Autodesk Fusion 360 part; units mm, degrees
(part 3 of 5)
extrude "Finger lift notch''''" cut sketch "草图17 (3)" along normal blind 4 bodies 10 in component "LS_RemovableGrate"
chamfer "R03 touch edge chamfer'''''''''" distance 0.4 angle 45 5 edges at (166.7, 184.65, 30) (110, 318.7, 30) (166.7, 279.35, 30) (110, 145.3, 30) (53.3, 232, 30) on bodies 10 in component "LS_RemovableGrate"
ref_plane "工作平面1" through (0, 0, 10) normal (0, 0, 1) x (1, 0, 0) in component "RS_Integrated"
sketch "草图1 (11)" plane through (0, 0, 10) normal (0, 0, 1) x (1, 0, 0) in component "RS_Integrated"
  line L0 (770, 142) -> (860, 142)
  line L1 (860, 142) -> (860, 322)
  line L2 (860, 322) -> (770, 322)
  line L3 (770, 322) -> (770, 142)
  dimension "d1020" = 770
  dimension "d1021" = 142
  dimension "d1022" = 90
  dimension "d1023" = 180
  constraint horizontal L0
  constraint vertical L1
  constraint horizontal L2
  constraint vertical L3
  measures "d1020" horizontal distance of origin L0.start
  measures "d1021" vertical distance of origin L0.start
  measures "d1022" horizontal distance of L0.start L0.end
  measures "d1023" vertical distance of L0.end L1.end
extrude "R04 pan blank'''''" add sketch "草图1 (11)" along normal blind 20 separate body makes body 11 in component "RS_Integrated"
fillet "Outside corner rounds'''''" radius 3 4 edges at (770, 322, 20) (860, 322, 20) (860, 142, 20) (770, 142, 20) on bodies 11 in component "RS_Integrated"
ref_plane "工作平面2" through (0, 145, 0) normal (0, 1, 0) x (0, 0, 1) in component "RS_Integrated"
sketch "草图2 (11)" plane through (0, 145, 0) normal (0, 1, 0) x (1, 0, 0) in component "RS_Integrated"
  line L0 (857, -22.1441) -> (770, -13)
  line L1 (770, -13) -> (770, -31)
  line L2 (770, -31) -> (857, -31)
  line L3 (857, -31) -> (857, -22.1441)
  dimension "d1030" = 857
  dimension "d1031" = 22.1441
  dimension "d1032" = 770
  dimension "d1033" = 13
  dimension "d1034" = 31
  constraint vertical L1
  constraint horizontal L2
  constraint vertical L3
  measures "d1030" horizontal distance of origin L0.start
  measures "d1031" vertical distance of origin L0.start
  measures "d1032" horizontal distance of origin L0.end
  measures "d1033" vertical distance of origin L0.end
  measures "d1034" vertical distance of origin L1.end
extrude "R04 continuous slope and open edge'''''" cut sketch "草图2 (11)" along normal blind 174 bodies 11 in component "RS_Integrated"
ref_plane "工作平面3" through (0, 0, 10) normal (0, 0, 1) x (1, 0, 0) in component "RS_Integrated"
sketch "草图3 (11)" plane through (0, 0, 10) normal (0, 0, 1) x (1, 0, 0) in component "RS_Integrated"
  line L0 (845, 145) -> (857, 145)
  line L1 (857, 145) -> (857, 157)
  line L2 (857, 157) -> (845, 157)
  line L3 (845, 157) -> (845, 145)
  dimension "d1039" = 845
  dimension "d1041" = 12
  dimension "d1042" = 12
  constraint horizontal L0
  constraint vertical L1
  constraint horizontal L2
  constraint vertical L3
  measures "d1039" horizontal distance of origin L0.start
  measures "d1041" horizontal distance of L0.start L0.end
  measures "d1042" vertical distance of L0.end L1.end
extrude "Grate seat 00'''''" add sketch "草图3 (11)" along normal blind 16 bodies 11 in component "RS_Integrated"
ref_plane "工作平面4" through (0, 0, 10) normal (0, 0, 1) x (1, 0, 0) in component "RS_Integrated"
sketch "草图4 (11)" plane through (0, 0, 10) normal (0, 0, 1) x (1, 0, 0) in component "RS_Integrated"
  line L0 (773, 145) -> (785, 145)
  line L1 (785, 145) -> (785, 157)
  line L2 (785, 157) -> (773, 157)
  line L3 (773, 157) -> (773, 145)
  dimension "d1047" = 773
  dimension "d1049" = 12
  dimension "d1050" = 12
  constraint horizontal L0
  constraint vertical L1
  constraint horizontal L2
  constraint vertical L3
  measures "d1047" horizontal distance of origin L0.start
  measures "d1049" horizontal distance of L0.start L0.end
  measures "d1050" vertical distance of L0.end L1.end
extrude "Grate seat 01'''''" add sketch "草图4 (11)" along normal blind 16 bodies 11 in component "RS_Integrated"
ref_plane "工作平面5" through (0, 0, 10) normal (0, 0, 1) x (1, 0, 0) in component "RS_Integrated"
sketch "草图5 (11)" plane through (0, 0, 10) normal (0, 0, 1) x (1, 0, 0) in component "RS_Integrated"
  line L0 (845, 307) -> (857, 307)
  line L1 (857, 307) -> (857, 319)
  line L2 (857, 319) -> (845, 319)
  line L3 (845, 319) -> (845, 307)
  dimension "d1055" = 845
  dimension "d1056" = 307
  dimension "d1057" = 12
  dimension "d1058" = 12
  constraint horizontal L0
  constraint vertical L1
  constraint horizontal L2
  constraint vertical L3
  measures "d1055" horizontal distance of origin L0.start
  measures "d1056" vertical distance of origin L0.start
  measures "d1057" horizontal distance of L0.start L0.end
  measures "d1058" vertical distance of L0.end L1.end
extrude "Grate seat 10'''''" add sketch "草图5 (11)" along normal blind 16 bodies 11 in component "RS_Integrated"
ref_plane "工作平面6" through (0, 0, 10) normal (0, 0, 1) x (1, 0, 0) in component "RS_Integrated"
sketch "草图6 (11)" plane through (0, 0, 10) normal (0, 0, 1) x (1, 0, 0) in component "RS_Integrated"
  line L0 (773, 307) -> (785, 307)
  line L1 (785, 307) -> (785, 319)
  line L2 (785, 319) -> (773, 319)
  line L3 (773, 319) -> (773, 307)
  dimension "d1063" = 773
  dimension "d1064" = 307
  dimension "d1065" = 12
  dimension "d1066" = 12
  constraint horizontal L0
  constraint vertical L1
  constraint horizontal L2
  constraint vertical L3
  measures "d1063" horizontal distance of origin L0.start
  measures "d1064" vertical distance of origin L0.start
  measures "d1065" horizontal distance of L0.start L0.end
  measures "d1066" vertical distance of L0.end L1.end
extrude "Grate seat 11'''''" add sketch "草图6 (11)" along normal blind 16 bodies 11 in component "RS_Integrated"
ref_plane "工作平面7" through (0, 0, 0) normal (0, 0, 1) x (1, 0, 0) in component "RS_Integrated"
sketch "草图7 (11)" plane through (0, 0, 0) normal (0, 0, 1) x (1, 0, 0) in component "RS_Integrated"
  line L0 (779, 145) -> (860, 145)
  line L1 (860, 145) -> (860, 153)
  line L2 (860, 153) -> (779, 153)
  line L3 (779, 153) -> (779, 145)
  dimension "d1071" = 779
  dimension "d1072" = 145
  dimension "d1073" = 81
  dimension "d1074" = 8
  constraint horizontal L0
  constraint vertical L1
  constraint horizontal L2
  constraint vertical L3
  measures "d1071" horizontal distance of origin L0.start
  measures "d1072" vertical distance of origin L0.start
  measures "d1073" horizontal distance of L0.start L0.end
  measures "d1074" vertical distance of L0.end L1.end
extrude "R04 low integral runner 0'''''" add sketch "草图7 (11)" along normal blind 10 bodies 11 in component "RS_Integrated"
ref_plane "工作平面8" through (0, 0, 0) normal (0, 0, 1) x (1, 0, 0) in component "RS_Integrated"
sketch "草图8 (11)" plane through (0, 0, 0) normal (0, 0, 1) x (1, 0, 0) in component "RS_Integrated"
  line L0 (779, 311) -> (860, 311)
  line L1 (860, 311) -> (860, 319)
  line L2 (860, 319) -> (779, 319)
  line L3 (779, 319) -> (779, 311)
  dimension "d1079" = 779
  dimension "d1080" = 311
  dimension "d1081" = 81
  dimension "d1082" = 8
  constraint horizontal L0
  constraint vertical L1
  constraint horizontal L2
  constraint vertical L3
  measures "d1079" horizontal distance of origin L0.start
  measures "d1080" vertical distance of origin L0.start
  measures "d1081" horizontal distance of L0.start L0.end
  measures "d1082" vertical distance of L0.end L1.end
extrude "R04 low integral runner 1'''''" add sketch "草图8 (11)" along normal blind 10 bodies 11 in component "RS_Integrated"
chamfer "R03 touch edge chamfer''''''''''" distance 0.4 angle 45 5 edges at (813.5, 145, 30) (813.5, 319, 30) (857, 232, 30) (815, 142, 30) (815, 322, 30) on bodies 11 in component "RS_Integrated"
ref_plane "工作平面1" through (0, 0, 26) normal (0, 0, 1) x (1, 0, 0) in component "RS_RemovableGrate"
sketch "草图1 (12)" plane through (0, 0, 26) normal (0, 0, 1) x (1, 0, 0) in component "RS_RemovableGrate"
  line L0 (773.3, 145.3) -> (856.7, 145.3)
  line L1 (856.7, 145.3) -> (856.7, 318.7)
  line L2 (856.7, 318.7) -> (773.3, 318.7)
  line L3 (773.3, 318.7) -> (773.3, 145.3)
  dimension "d1088" = 773.3
  dimension "d1090" = 83.4
  dimension "d1091" = 173.4
  constraint horizontal L0
  constraint vertical L1
  constraint horizontal L2
  constraint vertical L3
  measures "d1088" horizontal distance of origin L0.start
  measures "d1090" horizontal distance of L0.start L0.end
  measures "d1091" vertical distance of L0.end L1.end
extrude "Horizontal removable deck'''''" add sketch "草图1 (12)" along normal blind 4 separate body makes body 12 in component "RS_RemovableGrate"
ref_plane "工作平面2" through (0, 0, 26) normal (0, 0, 1) x (1, 0, 0) in component "RS_RemovableGrate"
sketch "草图2 (12)" plane through (0, 0, 26) normal (0, 0, 1) x (1, 0, 0) in component "RS_RemovableGrate"
  line L0 (780.3, 160) -> (849.7, 160)
  line L1 (849.7, 160) -> (849.7, 164)
  line L2 (849.7, 164) -> (780.3, 164)
  line L3 (780.3, 164) -> (780.3, 160)
  dimension "d1096" = 780.3
  dimension "d1097" = 160
  dimension "d1098" = 69.4
  dimension "d1099" = 4
  constraint horizontal L0
  constraint vertical L1
  constraint horizontal L2
  constraint vertical L3
  measures "d1096" horizontal distance of origin L0.start
  measures "d1097" vertical distance of origin L0.start
  measures "d1098" horizontal distance of L0.start L0.end
  measures "d1099" vertical distance of L0.end L1.end
extrude "Drain slot 1'''''" cut sketch "草图2 (12)" along normal blind 4 bodies 12 in component "RS_RemovableGrate"
ref_plane "工作平面3" through (0, 0, 26) normal (0, 0, 1) x (1, 0, 0) in component "RS_RemovableGrate"
sketch "草图3 (12)" plane through (0, 0, 26) normal (0, 0, 1) x (1, 0, 0) in component "RS_RemovableGrate"
  line L0 (780.3, 170) -> (849.7, 170)
  line L1 (849.7, 170) -> (849.7, 174)
  line L2 (849.7, 174) -> (780.3, 174)
  line L3 (780.3, 174) -> (780.3, 170)
  dimension "d1104" = 780.3
  dimension "d1105" = 170
  dimension "d1106" = 69.4
  dimension "d1107" = 4
  constraint horizontal L0
  constraint vertical L1
  constraint horizontal L2
  constraint vertical L3
  measures "d1104" horizontal distance of origin L0.start
  measures "d1105" vertical distance of origin L0.start
  measures "d1106" horizontal distance of L0.start L0.end
  measures "d1107" vertical distance of L0.end L1.end
extrude "Drain slot 2'''''" cut sketch "草图3 (12)" along normal blind 4 bodies 12 in component "RS_RemovableGrate"
ref_plane "工作平面4" through (0, 0, 26) normal (0, 0, 1) x (1, 0, 0) in component "RS_RemovableGrate"
sketch "草图4 (12)" plane through (0, 0, 26) normal (0, 0, 1) x (1, 0, 0) in component "RS_RemovableGrate"
  line L0 (780.3, 180) -> (849.7, 180)
  line L1 (849.7, 180) -> (849.7, 184)
  line L2 (849.7, 184) -> (780.3, 184)
  line L3 (780.3, 184) -> (780.3, 180)
  dimension "d1112" = 780.3
  dimension "d1113" = 180
  dimension "d1114" = 69.4
  dimension "d1115" = 4
  constraint horizontal L0
  constraint vertical L1
  constraint horizontal L2
  constraint vertical L3
  measures "d1112" horizontal distance of origin L0.start
  measures "d1113" vertical distance of origin L0.start
  measures "d1114" horizontal distance of L0.start L0.end
  measures "d1115" vertical distance of L0.end L1.end
extrude "Drain slot 3'''''" cut sketch "草图4 (12)" along normal blind 4 bodies 12 in component "RS_RemovableGrate"
ref_plane "工作平面5" through (0, 0, 26) normal (0, 0, 1) x (1, 0, 0) in component "RS_RemovableGrate"
sketch "草图5 (12)" plane through (0, 0, 26) normal (0, 0, 1) x (1, 0, 0) in component "RS_RemovableGrate"
  line L0 (780.3, 190) -> (849.7, 190)
  line L1 (849.7, 190) -> (849.7, 194)
  line L2 (849.7, 194) -> (780.3, 194)
  line L3 (780.3, 194) -> (780.3, 190)
  dimension "d1120" = 780.3
  dimension "d1121" = 190
  dimension "d1122" = 69.4
  dimension "d1123" = 4
  constraint horizontal L0
  constraint vertical L1
  constraint horizontal L2
  constraint vertical L3
  measures "d1120" horizontal distance of origin L0.start
  measures "d1121" vertical distance of origin L0.start
  measures "d1122" horizontal distance of L0.start L0.end
  measures "d1123" vertical distance of L0.end L1.end
extrude "Drain slot 4'''''" cut sketch "草图5 (12)" along normal blind 4 bodies 12 in component "RS_RemovableGrate"
ref_plane "工作平面6" through (0, 0, 26) normal (0, 0, 1) x (1, 0, 0) in component "RS_RemovableGrate"
sketch "草图6 (12)" plane through (0, 0, 26) normal (0, 0, 1) x (1, 0, 0) in component "RS_RemovableGrate"
  line L0 (780.3, 200) -> (849.7, 200)
  line L1 (849.7, 200) -> (849.7, 204)
  line L2 (849.7, 204) -> (780.3, 204)
  line L3 (780.3, 204) -> (780.3, 200)
  dimension "d1128" = 780.3
  dimension "d1129" = 200
  dimension "d1130" = 69.4
  dimension "d1131" = 4
  constraint horizontal L0
  constraint vertical L1
  constraint horizontal L2
  constraint vertical L3
  measures "d1128" horizontal distance of origin L0.start
  measures "d1129" vertical distance of origin L0.start
  measures "d1130" horizontal distance of L0.start L0.end
  measures "d1131" vertical distance of L0.end L1.end
extrude "Drain slot 5'''''" cut sketch "草图6 (12)" along normal blind 4 bodies 12 in component "RS_RemovableGrate"
ref_plane "工作平面7" through (0, 0, 26) normal (0, 0, 1) x (1, 0, 0) in component "RS_RemovableGrate"
sketch "草图7 (12)" plane through (0, 0, 26) normal (0, 0, 1) x (1, 0, 0) in component "RS_RemovableGrate"
  line L0 (780.3, 210) -> (849.7, 210)
  line L1 (849.7, 210) -> (849.7, 214)
  line L2 (849.7, 214) -> (780.3, 214)
  line L3 (780.3, 214) -> (780.3, 210)
  dimension "d1136" = 780.3
  dimension "d1137" = 210
  dimension "d1138" = 69.4
  dimension "d1139" = 4
  constraint horizontal L0
  constraint vertical L1
  constraint horizontal L2
  constraint vertical L3
  measures "d1136" horizontal distance of origin L0.start
  measures "d1137" vertical distance of origin L0.start
  measures "d1138" horizontal distance of L0.start L0.end
  measures "d1139" vertical distance of L0.end L1.end
extrude "Drain slot 6'''''" cut sketch "草图7 (12)" along normal blind 4 bodies 12 in component "RS_RemovableGrate"
ref_plane "工作平面8" through (0, 0, 26) normal (0, 0, 1) x (1, 0, 0) in component "RS_RemovableGrate"
sketch "草图8 (12)" plane through (0, 0, 26) normal (0, 0, 1) x (1, 0, 0) in component "RS_RemovableGrate"
  line L0 (780.3, 220) -> (849.7, 220)
  line L1 (849.7, 220) -> (849.7, 224)
  line L2 (849.7, 224) -> (780.3, 224)
  line L3 (780.3, 224) -> (780.3, 220)
  dimension "d1144" = 780.3
  dimension "d1145" = 220
  dimension "d1146" = 69.4
  dimension "d1147" = 4
  constraint horizontal L0
  constraint vertical L1
  constraint horizontal L2
  constraint vertical L3
  measures "d1144" horizontal distance of origin L0.start
  measures "d1145" vertical distance of origin L0.start
  measures "d1146" horizontal distance of L0.start L0.end
  measures "d1147" vertical distance of L0.end L1.end
extrude "Drain slot 7'''''" cut sketch "草图8 (12)" along normal blind 4 bodies 12 in component "RS_RemovableGrate"
ref_plane "工作平面9" through (0, 0, 26) normal (0, 0, 1) x (1, 0, 0) in component "RS_RemovableGrate"
sketch "草图9 (6)" plane through (0, 0, 26) normal (0, 0, 1) x (1, 0, 0) in component "RS_RemovableGrate"
  line L0 (780.3, 230) -> (849.7, 230)
  line L1 (849.7, 230) -> (849.7, 234)
  line L2 (849.7, 234) -> (780.3, 234)
  line L3 (780.3, 234) -> (780.3, 230)
  dimension "d1152" = 780.3
  dimension "d1153" = 230
  dimension "d1154" = 69.4
  dimension "d1155" = 4
  constraint horizontal L0
  constraint vertical L1
  constraint horizontal L2
  constraint vertical L3
  measures "d1152" horizontal distance of origin L0.start
  measures "d1153" vertical distance of origin L0.start
  measures "d1154" horizontal distance of L0.start L0.end
  measures "d1155" vertical distance of L0.end L1.end
extrude "Drain slot 8'''''" cut sketch "草图9 (6)" along normal blind 4 bodies 12 in component "RS_RemovableGrate"
ref_plane "工作平面10" through (0, 0, 26) normal (0, 0, 1) x (1, 0, 0) in component "RS_RemovableGrate"
sketch "草图10 (6)" plane through (0, 0, 26) normal (0, 0, 1) x (1, 0, 0) in component "RS_RemovableGrate"
  line L0 (780.3, 240) -> (849.7, 240)
  line L1 (849.7, 240) -> (849.7, 244)
  line L2 (849.7, 244) -> (780.3, 244)
  line L3 (780.3, 244) -> (780.3, 240)
  dimension "d1160" = 780.3
  dimension "d1161" = 240
  dimension "d1162" = 69.4
  dimension "d1163" = 4
  constraint horizontal L0
  constraint vertical L1
  constraint horizontal L2
  constraint vertical L3
  measures "d1160" horizontal distance of origin L0.start
  measures "d1161" vertical distance of origin L0.start
  measures "d1162" horizontal distance of L0.start L0.end
  measures "d1163" vertical distance of L0.end L1.end
extrude "Drain slot 9'''''" cut sketch "草图10 (6)" along normal blind 4 bodies 12 in component "RS_RemovableGrate"
ref_plane "工作平面11" through (0, 0, 26) normal (0, 0, 1) x (1, 0, 0) in component "RS_RemovableGrate"
sketch "草图11 (6)" plane through (0, 0, 26) normal (0, 0, 1) x (1, 0, 0) in component "RS_RemovableGrate"
  line L0 (780.3, 250) -> (849.7, 250)
  line L1 (849.7, 250) -> (849.7, 254)
  line L2 (849.7, 254) -> (780.3, 254)
  line L3 (780.3, 254) -> (780.3, 250)
  dimension "d1168" = 780.3
  dimension "d1169" = 250
  dimension "d1170" = 69.4
  dimension "d1171" = 4
  constraint horizontal L0
  constraint vertical L1
  constraint horizontal L2
  constraint vertical L3
  measures "d1168" horizontal distance of origin L0.start
  measures "d1169" vertical distance of origin L0.start
  measures "d1170" horizontal distance of L0.start L0.end
  measures "d1171" vertical distance of L0.end L1.end
extrude "Drain slot 10'''''" cut sketch "草图11 (6)" along normal blind 4 bodies 12 in component "RS_RemovableGrate"
ref_plane "工作平面12" through (0, 0, 26) normal (0, 0, 1) x (1, 0, 0) in component "RS_RemovableGrate"
sketch "草图12 (6)" plane through (0, 0, 26) normal (0, 0, 1) x (1, 0, 0) in component "RS_RemovableGrate"
  line L0 (780.3, 260) -> (849.7, 260)
  line L1 (849.7, 260) -> (849.7, 264)
  line L2 (849.7, 264) -> (780.3, 264)
  line L3 (780.3, 264) -> (780.3, 260)
  dimension "d1176" = 780.3
  dimension "d1177" = 260
  dimension "d1178" = 69.4
  dimension "d1179" = 4
  constraint horizontal L0
  constraint vertical L1
  constraint horizontal L2
  constraint vertical L3
  measures "d1176" horizontal distance of origin L0.start
  measures "d1177" vertical distance of origin L0.start
  measures "d1178" horizontal distance of L0.start L0.end
  measures "d1179" vertical distance of L0.end L1.end
extrude "Drain slot 11'''''" cut sketch "草图12 (6)" along normal blind 4 bodies 12 in component "RS_RemovableGrate"
ref_plane "工作平面13" through (0, 0, 26) normal (0, 0, 1) x (1, 0, 0) in component "RS_RemovableGrate"
sketch "草图13 (6)" plane through (0, 0, 26) normal (0, 0, 1) x (1, 0, 0) in component "RS_RemovableGrate"
  line L0 (780.3, 270) -> (849.7, 270)
  line L1 (849.7, 270) -> (849.7, 274)
  line L2 (849.7, 274) -> (780.3, 274)
  line L3 (780.3, 274) -> (780.3, 270)
  dimension "d1184" = 780.3
  dimension "d1185" = 270
  dimension "d1186" = 69.4
  dimension "d1187" = 4
  constraint horizontal L0
  constraint vertical L1
  constraint horizontal L2
  constraint vertical L3
  measures "d1184" horizontal distance of origin L0.start
  measures "d1185" vertical distance of origin L0.start
  measures "d1186" horizontal distance of L0.start L0.end
  measures "d1187" vertical distance of L0.end L1.end
extrude "Drain slot 12'''" cut sketch "草图13 (6)" along normal blind 4 bodies 12 in component "RS_RemovableGrate"
ref_plane "工作平面14" through (0, 0, 26) normal (0, 0, 1) x (1, 0, 0) in component "RS_RemovableGrate"
sketch "草图14 (4)" plane through (0, 0, 26) normal (0, 0, 1) x (1, 0, 0) in component "RS_RemovableGrate"
  line L0 (780.3, 280) -> (849.7, 280)
  line L1 (849.7, 280) -> (849.7, 284)
  line L2 (849.7, 284) -> (780.3, 284)
  line L3 (780.3, 284) -> (780.3, 280)
  dimension "d1192" = 780.3
  dimension "d1193" = 280
  dimension "d1194" = 69.4
  dimension "d1195" = 4
  constraint horizontal L0
  constraint vertical L1
  constraint horizontal L2
  constraint vertical L3
  measures "d1192" horizontal distance of origin L0.start
  measures "d1193" vertical distance of origin L0.start
  measures "d1194" horizontal distance of L0.start L0.end
  measures "d1195" vertical distance of L0.end L1.end
extrude "Drain slot 13'''" cut sketch "草图14 (4)" along normal blind 4 bodies 12 in component "RS_RemovableGrate"
ref_plane "工作平面15" through (0, 0, 26) normal (0, 0, 1) x (1, 0, 0) in component "RS_RemovableGrate"
sketch "草图15 (4)" plane through (0, 0, 26) normal (0, 0, 1) x (1, 0, 0) in component "RS_RemovableGrate"
  line L0 (780.3, 290) -> (849.7, 290)
  line L1 (849.7, 290) -> (849.7, 294)
  line L2 (849.7, 294) -> (780.3, 294)
  line L3 (780.3, 294) -> (780.3, 290)
  dimension "d1200" = 780.3
  dimension "d1201" = 290
  dimension "d1202" = 69.4
  dimension "d1203" = 4
  constraint horizontal L0
  constraint vertical L1
  constraint horizontal L2
  constraint vertical L3
  measures "d1200" horizontal distance of origin L0.start
  measures "d1201" vertical distance of origin L0.start
  measures "d1202" horizontal distance of L0.start L0.end
  measures "d1203" vertical distance of L0.end L1.end
extrude "Drain slot 14'''" cut sketch "草图15 (4)" along normal blind 4 bodies 12 in component "RS_RemovableGrate"
ref_plane "工作平面16" through (0, 0, 26) normal (0, 0, 1) x (1, 0, 0) in component "RS_RemovableGrate"
sketch "草图16 (4)" plane through (0, 0, 26) normal (0, 0, 1) x (1, 0, 0) in component "RS_RemovableGrate"
  line L0 (780.3, 300) -> (849.7, 300)
  line L1 (849.7, 300) -> (849.7, 304)
  line L2 (849.7, 304) -> (780.3, 304)
  line L3 (780.3, 304) -> (780.3, 300)
  dimension "d1208" = 780.3
  dimension "d1209" = 300
  dimension "d1210" = 69.4
  dimension "d1211" = 4
  constraint horizontal L0
  constraint vertical L1
  constraint horizontal L2
  constraint vertical L3
  measures "d1208" horizontal distance of origin L0.start
  measures "d1209" vertical distance of origin L0.start
  measures "d1210" horizontal distance of L0.start L0.end
  measures "d1211" vertical distance of L0.end L1.end
extrude "Drain slot 15'''" cut sketch "草图16 (4)" along normal blind 4 bodies 12 in component "RS_RemovableGrate"
ref_plane "工作平面17" through (0, 0, 26) normal (0, 0, 1) x (1, 0, 0) in component "RS_RemovableGrate"
sketch "草图17 (4)" plane through (0, 0, 26) normal (0, 0, 1) x (1, 0, 0) in component "RS_RemovableGrate"
  line L0 (772.3, 224) -> (777.3, 224)
  line L1 (777.3, 224) -> (777.3, 240)
  line L2 (777.3, 240) -> (772.3, 240)
  line L3 (772.3, 240) -> (772.3, 224)
  dimension "d1216" = 772.3
  dimension "d1217" = 224
  dimension "d1218" = 5
  dimension "d1219" = 16
  constraint horizontal L0
  constraint vertical L1
  constraint horizontal L2
  constraint vertical L3
  measures "d1216" horizontal distance of origin L0.start
  measures "d1217" vertical distance of origin L0.start
  measures "d1218" horizontal distance of L0.start L0.end
  measures "d1219" vertical distance of L0.end L1.end
extrude "Finger lift notch'''''" cut sketch "草图17 (4)" along normal blind 4 bodies 12 in component "RS_RemovableGrate"
chamfer "R03 touch edge chamfer'''''''''''" distance 0.4 angle 45 5 edges at (773.3, 184.65, 30) (815, 145.3, 30) (856.7, 232, 30) (815, 318.7, 30) (773.3, 279.35, 30) on bodies 12 in component "RS_RemovableGrate"
ref_plane "工作平面18" through (0, 0, 26) normal (0, 0, 1) x (1, 0, 0) in component "L1_RemovableGrate"
sketch "草图18 (2)" plane through (0, 0, 26) normal (0, 0, 1) x (1, 0, 0) in component "L1_RemovableGrate"
  line L0 (52.7, 59.7) -> (55.3, 59.7)
  line L1 (55.3, 59.7) -> (55.3, 65.3)
  line L2 (55.3, 65.3) -> (52.7, 65.3)
  line L3 (52.7, 65.3) -> (52.7, 59.7)
  dimension "d1226" = 59.7
  dimension "d1227" = 2.6
  dimension "d1228" = 5.6
  constraint horizontal L0
  constraint vertical L1
  constraint horizontal L2
  constraint vertical L3
  measures "d1226" vertical distance of origin L0.start
  measures "d1227" horizontal distance of L0.start L0.end
  measures "d1228" vertical distance of L0.end L1.end
extrude "R04 grate locating notch 0" cut sketch "草图18 (2)" along normal blind 4 bodies 4 in component "L1_RemovableGrate"
ref_plane "工作平面9" through (0, 0, 10) normal (0, 0, 1) x (1, 0, 0) in component "L1_Integrated"
sketch "草图9 (7)" plane through (0, 0, 10) normal (0, 0, 1) x (1, 0, 0) in component "L1_Integrated"
  line L0 (53, 60) -> (55, 60)
  line L1 (55, 60) -> (55, 65)
  line L2 (55, 65) -> (53, 65)
  line L3 (53, 65) -> (53, 60)
  dimension "d1234" = 60
  dimension "d1235" = 2
  dimension "d1236" = 5
  constraint horizontal L0
  constraint vertical L1
  constraint horizontal L2
  constraint vertical L3
  measures "d1234" vertical distance of origin L0.start
  measures "d1235" horizontal distance of L0.start L0.end
  measures "d1236" vertical distance of L0.end L1.end
extrude "R04 grate locating key 0" add sketch "草图9 (7)" along normal blind 20 bodies 3 in component "L1_Integrated"
ref_plane "工作平面19" through (0, 0, 26) normal (0, 0, 1) x (1, 0, 0) in component "L1_RemovableGrate"
sketch "草图19 (2)" plane through (0, 0, 26) normal (0, 0, 1) x (1, 0, 0) in component "L1_RemovableGrate"
  line L0 (224.7, 59.7) -> (227.3, 59.7)
  line L1 (227.3, 59.7) -> (227.3, 65.3)
  line L2 (227.3, 65.3) -> (224.7, 65.3)
  line L3 (224.7, 65.3) -> (224.7, 59.7)
  dimension "d1241" = 224.7
  dimension "d1242" = 59.7
  dimension "d1243" = 2.6
  dimension "d1244" = 5.6
  constraint horizontal L0
  constraint vertical L1
  constraint horizontal L2
  constraint vertical L3
  measures "d1241" horizontal distance of origin L0.start
  measures "d1242" vertical distance of origin L0.start
  measures "d1243" horizontal distance of L0.start L0.end
  measures "d1244" vertical distance of L0.end L1.end
extrude "R04 grate locating notch 1" cut sketch "草图19 (2)" along normal blind 4 bodies 4 in component "L1_RemovableGrate"
ref_plane "工作平面10" through (0, 0, 10) normal (0, 0, 1) x (1, 0, 0) in component "L1_Integrated"
sketch "草图10 (7)" plane through (0, 0, 10) normal (0, 0, 1) x (1, 0, 0) in component "L1_Integrated"
  line L0 (225, 60) -> (227, 60)
  line L1 (227, 60) -> (227, 65)
  line L2 (227, 65) -> (225, 65)
  line L3 (225, 65) -> (225, 60)
  dimension "d1249" = 225
  dimension "d1250" = 60
  dimension "d1251" = 2
  dimension "d1252" = 5
  constraint horizontal L0
  constraint vertical L1
  constraint horizontal L2
  constraint vertical L3
  measures "d1249" horizontal distance of origin L0.start
  measures "d1250" vertical distance of origin L0.start
  measures "d1251" horizontal distance of L0.start L0.end
  measures "d1252" vertical distance of L0.end L1.end
extrude "R04 grate locating key 1" add sketch "草图10 (7)" along normal blind 20 bodies 3 in component "L1_Integrated"
ref_plane "工作平面20" through (0, 0, 26) normal (0, 0, 1) x (1, 0, 0) in component "L2_RemovableGrate"
sketch "草图20" plane through (0, 0, 26) normal (0, 0, 1) x (1, 0, 0) in component "L2_RemovableGrate"
  line L0 (234.7, 59.7) -> (237.3, 59.7)
  line L1 (237.3, 59.7) -> (237.3, 65.3)
  line L2 (237.3, 65.3) -> (234.7, 65.3)
  line L3 (234.7, 65.3) -> (234.7, 59.7)
  dimension "d1258" = 59.7
  dimension "d1259" = 2.6
  dimension "d1260" = 5.6
  constraint horizontal L0
  constraint vertical L1
  constraint horizontal L2
  constraint vertical L3
  measures "d1258" vertical distance of origin L0.start
  measures "d1259" horizontal distance of L0.start L0.end
  measures "d1260" vertical distance of L0.end L1.end
extrude "R04 grate locating notch 0'" cut sketch "草图20" along normal blind 4 bodies 6 in component "L2_RemovableGrate"
ref_plane "工作平面9" through (0, 0, 10) normal (0, 0, 1) x (1, 0, 0) in component "L2_Integrated"
sketch "草图9 (8)" plane through (0, 0, 10) normal (0, 0, 1) x (1, 0, 0) in component "L2_Integrated"
  line L0 (235, 60) -> (237, 60)
  line L1 (237, 60) -> (237, 65)
  line L2 (237, 65) -> (235, 65)
  line L3 (235, 65) -> (235, 60)
  dimension "d1266" = 60
  dimension "d1267" = 2
  dimension "d1268" = 5
  constraint horizontal L0
  constraint vertical L1
  constraint horizontal L2
  constraint vertical L3
  measures "d1266" vertical distance of origin L0.start
  measures "d1267" horizontal distance of L0.start L0.end
  measures "d1268" vertical distance of L0.end L1.end
extrude "R04 grate locating key 0'" add sketch "草图9 (8)" along normal blind 20 bodies 5 in component "L2_Integrated"
ref_plane "工作平面21" through (0, 0, 26) normal (0, 0, 1) x (1, 0, 0) in component "L2_RemovableGrate"
sketch "草图21" plane through (0, 0, 26) normal (0, 0, 1) x (1, 0, 0) in component "L2_RemovableGrate"
  line L0 (424.7, 59.7) -> (427.3, 59.7)
  line L1 (427.3, 59.7) -> (427.3, 65.3)
  line L2 (427.3, 65.3) -> (424.7, 65.3)
  line L3 (424.7, 65.3) -> (424.7, 59.7)
  dimension "d1273" = 424.7
  dimension "d1274" = 59.7
  dimension "d1275" = 2.6
  dimension "d1276" = 5.6
  constraint horizontal L0
  constraint vertical L1
  constraint horizontal L2
  constraint vertical L3
  measures "d1273" horizontal distance of origin L0.start
  measures "d1274" vertical distance of origin L0.start
  measures "d1275" horizontal distance of L0.start L0.end
  measures "d1276" vertical distance of L0.end L1.end
extrude "R04 grate locating notch 1'" cut sketch "草图21" along normal blind 4 bodies 6 in component "L2_RemovableGrate"
ref_plane "工作平面10" through (0, 0, 10) normal (0, 0, 1) x (1, 0, 0) in component "L2_Integrated"
sketch "草图10 (8)" plane through (0, 0, 10) normal (0, 0, 1) x (1, 0, 0) in component "L2_Integrated"
  line L0 (425, 60) -> (427, 60)
  line L1 (427, 60) -> (427, 65)
  line L2 (427, 65) -> (425, 65)
  line L3 (425, 65) -> (425, 60)
  dimension "d1281" = 425
  dimension "d1282" = 60
  dimension "d1283" = 2
  dimension "d1284" = 5
  constraint horizontal L0
  constraint vertical L1
  constraint horizontal L2
  constraint vertical L3
  measures "d1281" horizontal distance of origin L0.start
  measures "d1282" vertical distance of origin L0.start
  measures "d1283" horizontal distance of L0.start L0.end
  measures "d1284" vertical distance of L0.end L1.end
extrude "R04 grate locating key 1'" add sketch "草图10 (8)" along normal blind 20 bodies 5 in component "L2_Integrated"
ref_plane "工作平面14" through (0, 0, 26) normal (0, 0, 1) x (1, 0, 0) in component "R1_RemovableGrate"
sketch "草图14 (5)" plane through (0, 0, 26) normal (0, 0, 1) x (1, 0, 0) in component "R1_RemovableGrate"
  line L0 (592.7, 59.7) -> (595.3, 59.7)
  line L1 (595.3, 59.7) -> (595.3, 65.3)
  line L2 (595.3, 65.3) -> (592.7, 65.3)
  line L3 (592.7, 65.3) -> (592.7, 59.7)
  dimension "d1290" = 59.7
  dimension "d1291" = 2.6
  dimension "d1292" = 5.6
  constraint horizontal L0
  constraint vertical L1
  constraint horizontal L2
  constraint vertical L3
  measures "d1290" vertical distance of origin L0.start
  measures "d1291" horizontal distance of L0.start L0.end
  measures "d1292" vertical distance of L0.end L1.end
extrude "R04 grate locating notch 0''" cut sketch "草图14 (5)" along normal blind 4 bodies 2 in component "R1_RemovableGrate"
ref_plane "工作平面9" through (0, 0, 10) normal (0, 0, 1) x (1, 0, 0) in component "R1_Integrated"
sketch "草图9 (9)" plane through (0, 0, 10) normal (0, 0, 1) x (1, 0, 0) in component "R1_Integrated"
  line L0 (593, 60) -> (595, 60)
  line L1 (595, 60) -> (595, 65)
  line L2 (595, 65) -> (593, 65)
  line L3 (593, 65) -> (593, 60)
  dimension "d1298" = 60
  dimension "d1299" = 2
  dimension "d1300" = 5
  constraint horizontal L0
  constraint vertical L1
  constraint horizontal L2
  constraint vertical L3
  measures "d1298" vertical distance of origin L0.start
  measures "d1299" horizontal distance of L0.start L0.end
  measures "d1300" vertical distance of L0.end L1.end
extrude "R04 grate locating key 0''" add sketch "草图9 (9)" along normal blind 20 bodies 1 in component "R1_Integrated"
ref_plane "工作平面15" through (0, 0, 26) normal (0, 0, 1) x (1, 0, 0) in component "R1_RemovableGrate"
sketch "草图15 (5)" plane through (0, 0, 26) normal (0, 0, 1) x (1, 0, 0) in component "R1_RemovableGrate"
  line L0 (718.7, 59.7) -> (721.3, 59.7)
  line L1 (721.3, 59.7) -> (721.3, 65.3)
  line L2 (721.3, 65.3) -> (718.7, 65.3)
  line L3 (718.7, 65.3) -> (718.7, 59.7)
  dimension "d1305" = 718.7
  dimension "d1306" = 59.7
  dimension "d1307" = 2.6
  dimension "d1308" = 5.6
  constraint horizontal L0
  constraint vertical L1
  constraint horizontal L2
  constraint vertical L3
  measures "d1305" horizontal distance of origin L0.start
  measures "d1306" vertical distance of origin L0.start
  measures "d1307" horizontal distance of L0.start L0.end
  measures "d1308" vertical distance of L0.end L1.end
extrude "R04 grate locating notch 1''" cut sketch "草图15 (5)" along normal blind 4 bodies 2 in component "R1_RemovableGrate"
ref_plane "工作平面10" through (0, 0, 10) normal (0, 0, 1) x (1, 0, 0) in component "R1_Integrated"
sketch "草图10 (9)" plane through (0, 0, 10) normal (0, 0, 1) x (1, 0, 0) in component "R1_Integrated"
  line L0 (719, 60) -> (721, 60)
  line L1 (721, 60) -> (721, 65)
  line L2 (721, 65) -> (719, 65)
  line L3 (719, 65) -> (719, 60)
  dimension "d1313" = 719
  dimension "d1314" = 60
  dimension "d1315" = 2
  dimension "d1316" = 5
  constraint horizontal L0
  constraint vertical L1
  constraint horizontal L2
  constraint vertical L3
  measures "d1313" horizontal distance of origin L0.start
  measures "d1314" vertical distance of origin L0.start
  measures "d1315" horizontal distance of L0.start L0.end
  measures "d1316" vertical distance of L0.end L1.end
extrude "R04 grate locating key 1''" add sketch "草图10 (9)" along normal blind 20 bodies 1 in component "R1_Integrated"
ref_plane "工作平面14" through (0, 0, 26) normal (0, 0, 1) x (1, 0, 0) in component "R2_RemovableGrate"
sketch "草图14 (6)" plane through (0, 0, 26) normal (0, 0, 1) x (1, 0, 0) in component "R2_RemovableGrate"
  line L0 (728.7, 59.7) -> (731.3, 59.7)
  line L1 (731.3, 59.7) -> (731.3, 65.3)
  line L2 (731.3, 65.3) -> (728.7, 65.3)
  line L3 (728.7, 65.3) -> (728.7, 59.7)
  dimension "d1321" = 728.7
  dimension "d1322" = 59.7
  dimension "d1323" = 2.6
  dimension "d1324" = 5.6
  constraint horizontal L0
  constraint vertical L1
  constraint horizontal L2
  constraint vertical L3
  measures "d1321" horizontal distance of origin L0.start
  measures "d1322" vertical distance of origin L0.start
  measures "d1323" horizontal distance of L0.start L0.end
  measures "d1324" vertical distance of L0.end L1.end
extrude "R04 grate locating notch 0'''" cut sketch "草图14 (6)" along normal blind 4 bodies 8 in component "R2_RemovableGrate"
ref_plane "工作平面9" through (0, 0, 10) normal (0, 0, 1) x (1, 0, 0) in component "R2_Integrated"
sketch "草图9 (10)" plane through (0, 0, 10) normal (0, 0, 1) x (1, 0, 0) in component "R2_Integrated"
  line L0 (729, 60) -> (731, 60)
  line L1 (731, 60) -> (731, 65)
  line L2 (731, 65) -> (729, 65)
  line L3 (729, 65) -> (729, 60)
  dimension "d1329" = 729
  dimension "d1330" = 60
  dimension "d1331" = 2
  dimension "d1332" = 5
  constraint horizontal L0
  constraint vertical L1
  constraint horizontal L2
  constraint vertical L3
  measures "d1329" horizontal distance of origin L0.start
  measures "d1330" vertical distance of origin L0.start
  measures "d1331" horizontal distance of L0.start L0.end
  measures "d1332" vertical distance of L0.end L1.end
extrude "R04 grate locating key 0'''" add sketch "草图9 (10)" along normal blind 20 bodies 7 in component "R2_Integrated"
ref_plane "工作平面15" through (0, 0, 26) normal (0, 0, 1) x (1, 0, 0) in component "R2_RemovableGrate"
sketch "草图15 (6)" plane through (0, 0, 26) normal (0, 0, 1) x (1, 0, 0) in component "R2_RemovableGrate"
  line L0 (854.7, 59.7) -> (857.3, 59.7)
  line L1 (857.3, 59.7) -> (857.3, 65.3)
  line L2 (857.3, 65.3) -> (854.7, 65.3)
  line L3 (854.7, 65.3) -> (854.7, 59.7)
  dimension "d1337" = 854.7
  dimension "d1338" = 59.7
  dimension "d1339" = 2.6
  dimension "d1340" = 5.6
  constraint horizontal L0
  constraint vertical L1
  constraint horizontal L2
  constraint vertical L3
  measures "d1337" horizontal distance of origin L0.start
  measures "d1338" vertical distance of origin L0.start
  measures "d1339" horizontal distance of L0.start L0.end
  measures "d1340" vertical distance of L0.end L1.end
extrude "R04 grate locating notch 1'''" cut sketch "草图15 (6)" along normal blind 4 bodies 8 in component "R2_RemovableGrate"
ref_plane "工作平面10" through (0, 0, 10) normal (0, 0, 1) x (1, 0, 0) in component "R2_Integrated"
sketch "草图10 (10)" plane through (0, 0, 10) normal (0, 0, 1) x (1, 0, 0) in component "R2_Integrated"
  line L0 (855, 60) -> (857, 60)
  line L1 (857, 60) -> (857, 65)
  line L2 (857, 65) -> (855, 65)
  line L3 (855, 65) -> (855, 60)
  dimension "d1345" = 855
  dimension "d1346" = 60
  dimension "d1347" = 2
  dimension "d1348" = 5
  constraint horizontal L0
  constraint vertical L1
  constraint horizontal L2
  constraint vertical L3
  measures "d1345" horizontal distance of origin L0.start
  measures "d1346" vertical distance of origin L0.start
  measures "d1347" horizontal distance of L0.start L0.end
  measures "d1348" vertical distance of L0.end L1.end
extrude "R04 grate locating key 1'''" add sketch "草图10 (10)" along normal blind 20 bodies 7 in component "R2_Integrated"
ref_plane "工作平面18" through (0, 0, 26) normal (0, 0, 1) x (1, 0, 0) in component "LS_RemovableGrate"
sketch "草图18 (3)" plane through (0, 0, 26) normal (0, 0, 1) x (1, 0, 0) in component "LS_RemovableGrate"
  line L0 (59.7, 316.7) -> (65.3, 316.7)
  line L1 (65.3, 316.7) -> (65.3, 319.3)
  line L2 (65.3, 319.3) -> (59.7, 319.3)
  line L3 (59.7, 319.3) -> (59.7, 316.7)
  dimension "d1353" = 59.7
  dimension "d1354" = 316.7
  dimension "d1355" = 5.6
  dimension "d1356" = 2.6
  constraint horizontal L0
  constraint vertical L1
  constraint horizontal L2
  constraint vertical L3
  measures "d1353" horizontal distance of origin L0.start
  measures "d1354" vertical distance of origin L0.start
  measures "d1355" horizontal distance of L0.start L0.end
  measures "d1356" vertical distance of L0.end L1.end
extrude "R04 grate locating notch 0''''" cut sketch "草图18 (3)" along normal blind 4 bodies 10 in component "LS_RemovableGrate"
ref_plane "工作平面9" through (0, 0, 10) normal (0, 0, 1) x (1, 0, 0) in component "LS_Integrated"
sketch "草图9 (11)" plane through (0, 0, 10) normal (0, 0, 1) x (1, 0, 0) in component "LS_Integrated"
  line L0 (60, 317) -> (65, 317)
  line L1 (65, 317) -> (65, 319)
  line L2 (65, 319) -> (60, 319)
  line L3 (60, 319) -> (60, 317)
  dimension "d1361" = 60
  dimension "d1362" = 317
  dimension "d1363" = 5
  dimension "d1364" = 2
  constraint horizontal L0
  constraint vertical L1
  constraint horizontal L2
  constraint vertical L3
  measures "d1361" horizontal distance of origin L0.start
  measures "d1362" vertical distance of origin L0.start
  measures "d1363" horizontal distance of L0.start L0.end
  measures "d1364" vertical distance of L0.end L1.end
extrude "R04 grate locating key 0''''" add sketch "草图9 (11)" along normal blind 20 bodies 9 in component "LS_Integrated"
ref_plane "工作平面19" through (0, 0, 26) normal (0, 0, 1) x (1, 0, 0) in component "LS_RemovableGrate"
sketch "草图19 (3)" plane through (0, 0, 26) normal (0, 0, 1) x (1, 0, 0) in component "LS_RemovableGrate"
  line L0 (59.7, 144.7) -> (65.3, 144.7)
  line L1 (65.3, 144.7) -> (65.3, 147.3)
  line L2 (65.3, 147.3) -> (59.7, 147.3)
  line L3 (59.7, 147.3) -> (59.7, 144.7)
  dimension "d1369" = 59.7
  dimension "d1370" = 144.7
  dimension "d1371" = 5.6
  dimension "d1372" = 2.6
  constraint horizontal L0
  constraint vertical L1
  constraint horizontal L2
  constraint vertical L3
  measures "d1369" horizontal distance of origin L0.start
  measures "d1370" vertical distance of origin L0.start
  measures "d1371" horizontal distance of L0.start L0.end
  measures "d1372" vertical distance of L0.end L1.end
extrude "R04 grate locating notch 1''''" cut sketch "草图19 (3)" along normal blind 4 bodies 10 in component "LS_RemovableGrate"
ref_plane "工作平面10" through (0, 0, 10) normal (0, 0, 1) x (1, 0, 0) in component "LS_Integrated"
sketch "草图10 (11)" plane through (0, 0, 10) normal (0, 0, 1) x (1, 0, 0) in component "LS_Integrated"
  line L0 (60, 145) -> (65, 145)
  line L1 (65, 145) -> (65, 147)
  line L2 (65, 147) -> (60, 147)
  line L3 (60, 147) -> (60, 145)
  dimension "d1377" = 60
  dimension "d1378" = 145
  dimension "d1379" = 5
  dimension "d1380" = 2
  constraint horizontal L0
  constraint vertical L1
  constraint horizontal L2
  constraint vertical L3
  measures "d1377" horizontal distance of origin L0.start
  measures "d1378" vertical distance of origin L0.start
  measures "d1379" horizontal distance of L0.start L0.end
  measures "d1380" vertical distance of L0.end L1.end
extrude "R04 grate locating key 1''''" add sketch "草图10 (11)" along normal blind 20 bodies 9 in component "LS_Integrated"
ref_plane "工作平面18" through (0, 0, 26) normal (0, 0, 1) x (1, 0, 0) in component "RS_RemovableGrate"
sketch "草图18 (4)" plane through (0, 0, 26) normal (0, 0, 1) x (1, 0, 0) in component "RS_RemovableGrate"
  line L0 (844.7, 144.7) -> (850.3, 144.7)
  line L1 (850.3, 144.7) -> (850.3, 147.3)
  line L2 (850.3, 147.3) -> (844.7, 147.3)
  line L3 (844.7, 147.3) -> (844.7, 144.7)
  dimension "d1385" = 844.7
  dimension "d1387" = 5.6
  dimension "d1388" = 2.6
  constraint horizontal L0
  constraint vertical L1
  constraint horizontal L2
  constraint vertical L3
  measures "d1385" horizontal distance of origin L0.start
  measures "d1387" horizontal distance of L0.start L0.end
  measures "d1388" vertical distance of L0.end L1.end
extrude "R04 grate locating notch 0'''''" cut sketch "草图18 (4)" along normal blind 4 bodies 12 in component "RS_RemovableGrate"
ref_plane "工作平面9" through (0, 0, 10) normal (0, 0, 1) x (1, 0, 0) in component "RS_Integrated"
sketch "草图9 (12)" plane through (0, 0, 10) normal (0, 0, 1) x (1, 0, 0) in component "RS_Integrated"
  line L0 (845, 145) -> (850, 145)
  line L1 (850, 145) -> (850, 147)
  line L2 (850, 147) -> (845, 147)
  line L3 (845, 147) -> (845, 145)
  dimension "d1393" = 845
  dimension "d1395" = 5
  dimension "d1396" = 2
  constraint horizontal L0
  constraint vertical L1
  constraint horizontal L2
  constraint vertical L3
  measures "d1393" horizontal distance of origin L0.start
  measures "d1395" horizontal distance of L0.start L0.end
  measures "d1396" vertical distance of L0.end L1.end
extrude "R04 grate locating key 0'''''" add sketch "草图9 (12)" along normal blind 20 bodies 11 in component "RS_Integrated"
ref_plane "工作平面19" through (0, 0, 26) normal (0, 0, 1) x (1, 0, 0) in component "RS_RemovableGrate"
sketch "草图19 (4)" plane through (0, 0, 26) normal (0, 0, 1) x (1, 0, 0) in component "RS_RemovableGrate"
  line L0 (844.7, 316.7) -> (850.3, 316.7)
  line L1 (850.3, 316.7) -> (850.3, 319.3)
  line L2 (850.3, 319.3) -> (844.7, 319.3)
  line L3 (844.7, 319.3) -> (844.7, 316.7)
  dimension "d1401" = 844.7
  dimension "d1402" = 316.7
  dimension "d1403" = 5.6
  dimension "d1404" = 2.6
  constraint horizontal L0
  constraint vertical L1
  constraint horizontal L2
  constraint vertical L3
  measures "d1401" horizontal distance of origin L0.start
  measures "d1402" vertical distance of origin L0.start
  measures "d1403" horizontal distance of L0.start L0.end
  measures "d1404" vertical distance of L0.end L1.end
extrude "R04 grate locating notch 1'''''" cut sketch "草图19 (4)" along normal blind 4 bodies 12 in component "RS_RemovableGrate"
ref_plane "工作平面10" through (0, 0, 10) normal (0, 0, 1) x (1, 0, 0) in component "RS_Integrated"
sketch "草图10 (12)" plane through (0, 0, 10) normal (0, 0, 1) x (1, 0, 0) in component "RS_Integrated"
  line L0 (845, 317) -> (850, 317)
  line L1 (850, 317) -> (850, 319)
  line L2 (850, 319) -> (845, 319)
  line L3 (845, 319) -> (845, 317)
  dimension "d1409" = 845
  dimension "d1410" = 317
  dimension "d1411" = 5
  dimension "d1412" = 2
  constraint horizontal L0
  constraint vertical L1
  constraint horizontal L2
  constraint vertical L3
  measures "d1409" horizontal distance of origin L0.start
  measures "d1410" vertical distance of origin L0.start
  measures "d1411" horizontal distance of L0.start L0.end
  measures "d1412" vertical distance of L0.end L1.end
extrude "R04 grate locating key 1'''''" add sketch "草图10 (12)" along normal blind 20 bodies 11 in component "RS_Integrated"
component "R1_Integrated" placed x (1, 0, 0) y (0, 1, 0) z (0, 0, 1) at (0, 0, 0)
component "R1_RemovableGrate" placed x (1, 0, 0) y (0, 1, 0) z (0, 0, 1) at (0, 0, 0)
component "L1_Integrated" placed x (1, 0, 0) y (0, 1, 0) z (0, 0, 1) at (0, 0, 0)
component "L1_RemovableGrate" placed x (1, 0, 0) y (0, 1, 0) z (0, 0, 1) at (0, 0, 0)
component "L2_Integrated" placed x (1, 0, 0) y (0, 1, 0) z (0, 0, 1) at (0, 0, 0)
component "L2_RemovableGrate" placed x (1, 0, 0) y (0, 1, 0) z (0, 0, 1) at (0, 0, 0)
component "R2_Integrated" placed x (1, 0, 0) y (0, 1, 0) z (0, 0, 1) at (0, 0, 0)
component "R2_RemovableGrate" placed x (1, 0, 0) y (0, 1, 0) z (0, 0, 1) at (0, 0, 0)
component "LS_Integrated" placed x (1, 0, 0) y (0, 1, 0) z (0, 0, 1) at (0, 0, 0)
component "LS_RemovableGrate" placed x (1, 0, 0) y (0, 1, 0) z (0, 0, 1) at (0, 0, 0)
component "RS_Integrated" placed x (1, 0, 0) y (0, 1, 0) z (0, 0, 1) at (0, 0, 0)
component "RS_RemovableGrate" placed x (1, 0, 0) y (0, 1, 0) z (0, 0, 1) at (0, 0, 0)
equation "LeftAvailable = 400 mm" comment "User approximate dimension: left of faucet"
equation "RightAvailable = 300 mm" comment "User approximate dimension: right of faucet"
equation "RearAvailable = 100 mm" comment "User approximate rear strip depth"
equation "LeftSideAvailable = 130 mm" comment "User approximate left strip width"
equation "MirrorClearance = 300 mm" comment "User approximate countertop to mirror cabinet"
equation "RightSideAvailable = 100 mm" comment "ASSUMPTION: awaiting measurement"
equation "LeftReach = 180 mm" comment "ASSUMPTION: forward side extension beyond rear rack"
equation "RightReach = 180 mm" comment "ASSUMPTION: forward side extension beyond rear rack"
equation "FaucetGap = 160 mm" comment "ASSUMPTION: faucet and lever clearance, awaiting measurement"
equation "LeftRun = LeftAvailable - 20 mm" comment "Design clearance allowance; check on site"
equation "RightRun = RightAvailable - 30 mm" comment "Design clearance allowance; check lever"
equation "Depth = RearAvailable - 10 mm" comment "Rear standing module depth"
equation "LeftSideDepth = LeftSideAvailable - 10 mm" comment "Left side module depth"
equation "RightSideDepth = RightSideAvailable - 10 mm" comment "Right side module depth, provisional"
equation "ModuleGap = 2 mm" comment "Open cleaning / assembly seam, not watertight"
equation "TowerWidth = 180 mm" comment "Local upper tier only"
equation "TowerFrame = 8 mm" comment "Side portal frame thickness"
equation "TowerClearance = 2 mm" comment "Clearance from lower tray to side frames"
equation "FootHeight = 10 mm" comment "Clear gap below pan"
equation "PanHeight = 20 mm" comment "Pan rim above underside"
equation "FloorMin = 3 mm" comment "Minimum pan floor at outlet"
equation "Wall = 3 mm" comment "Pan walls"
equation "DrainSlope = 6 deg" comment "Initial design slope; verify with water test"
equation "DeckThick = 4 mm" comment "Removable horizontal grate thickness"
equation "DeckClearance = 0.3 mm" comment "Per-side clearance; fit coupon required"
equation "RimBorder = 7 mm" comment "Solid grate border"
equation "SlotWidth = 4 mm" comment "Open slat gaps"
equation "SlotPitch = 10 mm" comment "Initial grate slot spacing"
equation "DrainWidth = 28 mm" comment "R01 construction history only: R02 opens the entire front between side walls"
equation "DrainExtension = 0 mm" comment "R04 no projection and no inherited thickness offset"
equation "UpperDeckHeight = 145 mm" comment "Small jars only; verify cabinet swing"
equation "FootSize = 16 mm" comment "Support foot footprint"
equation "PegSize = 8 mm" comment "Square locating peg"
equation "PegHeight = 1.5 mm" comment "Foot locating peg, not a locking fastener"
equation "FitClearance = 0.25 mm" comment "Per-side foot fit allowance; test first"
equation "BaseX = 50 mm" comment "Model datum offset"
equation "BaseY = 50 mm" comment "Model datum offset"
equation "FrontFootInset = 17 mm" comment "R02 front foot center inset; outer foot edge is 9 mm behind open lip"
equation "TouchChamfer = 0.4 mm" comment "R03 selected touch edges; excludes drainage lip and locator bearing faces"
equation "RunnerWidth = 8 mm" comment "R03 integral support rail thickness"
equation "d41 = FootHeight"
equation "d43 = ( BaseX + LeftRun + FaucetGap ) + ( 0 mm )"
equation "d44 = ( BaseY ) + ( 0 mm )"
equation "d45 = ( RightRun - ModuleGap ) / 2"
equation "d46 = Depth"
equation "d47 = PanHeight"
equation "d51 = ( BaseX + LeftRun + FaucetGap ) + ( Wall )"
equation "d53 = -( -( ( FootHeight ) + FloorMin + ( ( Depth ) - ( Wall ) ) * tan(DrainSlope) ) )"
equation "d54 = ( ( BaseY ) + ( Wall ) )"
equation "d55 = -( -( ( FootHeight ) + FloorMin + ( ( Depth ) - ( Depth ) ) * tan(DrainSlope) ) )"
equation "d56 = ( ( BaseY ) + ( Depth ) )"
equation "d57 = -( -( FootHeight + PanHeight + 1 mm ) )"
equation "d58 = ( ( RightRun - ModuleGap ) / 2 ) - 2 * Wall"
equation "d60 = FootHeight"
equation "d62 = ( BaseX + LeftRun + FaucetGap ) + ( Wall )"
equation "d63 = ( BaseY ) + ( Wall )"
equation "d66 = PanHeight - DeckThick"
equation "d68 = FootHeight"
equation "d70 = ( BaseX + LeftRun + FaucetGap ) + ( Wall )"
equation "d71 = ( BaseY ) + ( ( Depth ) - Wall - 12 mm )"
equation "d74 = PanHeight - DeckThick"
equation "d76 = FootHeight"
equation "d78 = ( BaseX + LeftRun + FaucetGap ) + ( ( ( RightRun - ModuleGap ) / 2 ) - Wall - 12 mm )"
equation "d79 = ( BaseY ) + ( Wall )"
equation "d82 = PanHeight - DeckThick"